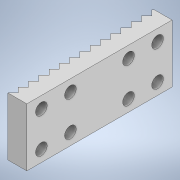
# Autodesk Inventor part: beltTensionerSide
Saved by Autodesk Inventor 2020 (Build 240168000, 168)
## iProperties
Created: 2020-01-19
Part Number: beltTensionerSide
Material: Generic
Document SubType Name: Modeling
Designer: PAB
Density: 1 g/cm^3
Appearance: Default
Author: PAB
Autodesk Inventor part; units mm, degrees
ref_plane "YZ Plane" through (0, 0, 0) normal (1, 0, 0) x (0, 1, 0)
ref_plane "XZ Plane" through (0, 0, 0) normal (0, 1, 0) x (-1, 0, 0)
ref_plane "XY Plane" through (0, 0, 0) normal (0, 0, 1) x (1, 0, 0)
sketch "Sketch1" plane through (0, 0, 0) normal (0, 1, 0) x (-1, 0, 0)
  line L0 (2, 25) -> (-2, 25)
  line L1 (-2, 25) -> (-2, -25)
  line L2 (-2, -25) -> (2, -25)
  line L3 (2, -25) -> (2, 25)
  line L4 (2, 25) -> (4.5, 25)
  line L5 (4.5, 25) -> (2.7322, 23.2322)
  line L6 (2.7322, 23.2322) -> (4.5, 21.4645)
  line L7 (4.5, 21.4645) -> (2.7322, 19.6967)
  line L8 (2.7322, 19.6967) -> (4.5, 17.9289)
  line L9 (4.5, 17.9289) -> (2.7322, 16.1612)
  line L10 (2.7322, 16.1612) -> (4.5, 14.3934)
  line L11 (4.5, 14.3934) -> (2.7322, 12.6256)
  line L12 (2.7322, 12.6256) -> (4.5, 10.8579)
  line L13 (4.5, 10.8579) -> (2.7322, 9.0901)
  line L14 (2.7322, 9.0901) -> (4.5, 7.3223)
  line L15 (4.5, 7.3223) -> (2.7322, 5.5546)
  line L16 (2.7322, 5.5546) -> (4.5, 3.7868)
  line L17 (4.5, 3.7868) -> (2.7322, 2.019)
  line L18 (2.7322, 2.019) -> (4.5, 0.2513)
  line L19 (4.5, 0.2513) -> (2.7322, -1.5165)
  line L20 (2.7322, -1.5165) -> (4.5, -3.2843)
  line L21 (4.5, -3.2843) -> (2.7322, -5.052)
  line L22 (2.7322, -5.052) -> (4.5, -6.8198)
  line L23 (4.5, -6.8198) -> (2.7322, -8.5876)
  line L24 (2.7322, -8.5876) -> (4.5, -10.3553)
  line L25 (4.5, -10.3553) -> (2.7322, -12.1231)
  line L26 (2.7322, -12.1231) -> (4.5, -13.8909)
  line L27 (4.5, -13.8909) -> (2.7322, -15.6586)
  line L28 (2.7322, -15.6586) -> (4.5, -17.4264)
  line L29 (4.5, -17.4264) -> (2.7322, -19.1942)
  line L30 (2.7322, -19.1942) -> (4.5, -20.9619)
  line L31 (4.5, -20.9619) -> (2.7322, -22.7297)
  line L32 (2.7322, -22.7297) -> (4.5, -24.4975)
  line L33 (4.5, -24.4975) -> (3.9975, -25)
  line L34 (3.9975, -25) -> (2, -25)
  point P0 (0, 0)
  dimension "d0" = 4
  dimension "d1" = 50
  dimension "d2" = 2.5
  dimension "d3" = 2.5
  dimension "d4" = 45
  dimension "d5" = 2.5
  constraints: 70 end point, 29 perpendicular, 2 horizontal, 2 parallel, 1 collinear
  measures "d0" distance of L2.end L1.end
  measures "d1" distance of L1.end L0.end
  measures "d2" distance of L0.start L4.end
  measures "d3" distance of L4.end L5.end
  measures "d4" angle of L4 L5
  measures "d5" distance of L5.end L6.end
extrude "Extrusion1" add sketch "Sketch1" along normal blind 20
sketch "Sketch2" plane through (2, 0, 25) normal (1, 0, 0) x (0, 0, -1)
  circle A0 centre (15, 4) radius 2
  circle A1 centre (35, 4) radius 2
  circle A2 centre (35, 16) radius 2
  circle A3 centre (15, 16) radius 2
  circle A4 centre (45, 16) radius 2
  circle A5 centre (45, 4) radius 2
  circle A6 centre (5, 4) radius 2
  circle A7 centre (5, 16) radius 2
  point P0 (25, 0)
  dimension "d8" = 4
  dimension "d9" = 4
  dimension "d10" = 4
  dimension "d11" = 4
  dimension "d12" = 4
  dimension "d13" = 4
  dimension "d14" = 4
  dimension "d15" = 4
  constraints: 8 centre point
  measures "d8" diameter of A0
  measures "d9" diameter of A1
  measures "d10" diameter of A2
  measures "d11" diameter of A3
  measures "d12" diameter of A4
  measures "d13" diameter of A5
  measures "d14" diameter of A6
  measures "d15" diameter of A7
extrude "Extrusion2" cut sketch "Sketch2" against normal blind 20
body "Solid1"
